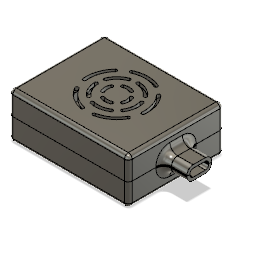
GBIP-uno (Autodesk Fusion 360 design; units mm, degrees)
Autodesk Fusion 360 part; units mm, degrees
sketch "Sketch1" plane through (0, 0, 0) normal (0, 1, 0) x (1, 0, 0)
  line L0 (0, 53.2694) -> (68.6417, 53.2694)
  line L1 (68.6417, 53.2694) -> (68.6417, 0.0072)
  line L2 (68.6417, 0.0072) -> (0, 0.0072)
  line L3 (0, 0.0072) -> (0, 53.2694)
  line L4 (70.6417, -1.9928) -> (-2, -1.9928)
  line L5 (-2, -1.9928) -> (-2, 55.2694)
  line L6 (-2, 55.2694) -> (70.6417, 55.2694)
  line L7 (70.6417, 55.2694) -> (70.6417, -1.9928)
  line L8 (70.1417, -4.4928) -> (-1.5, -4.4928)
  line L9 (-4.5, -1.4928) -> (-4.5, 54.7694)
  line L10 (-1.5, 57.7694) -> (70.1417, 57.7694)
  line L11 (73.1417, 54.7694) -> (73.1417, -1.4928)
  arc A0 (-1.5, 57.7694) -> (-4.5, 54.7694) centre (-1.5, 54.7694) ccw
  arc A1 (73.1417, 54.7694) -> (70.1417, 57.7694) centre (70.1417, 54.7694) ccw
  arc A2 (70.1417, -4.4928) -> (73.1417, -1.4928) centre (70.1417, -1.4928) ccw
  arc A3 (-4.5, -1.4928) -> (-1.5, -4.4928) centre (-1.5, -1.4928) ccw
  line L12 (11.9, 3.5) -> (0, 3.5)
  line L13 (0, 3.5) -> (0, 0)
  line L14 (0, 0) -> (66.1, 0)
  line L15 (66.1, 0) -> (66.1, 2)
  line L16 (66.1, 2) -> (68.6, 4.5)
  line L17 (68.6, 4.5) -> (68.6, 37.8)
  line L18 (68.6, 37.8) -> (66.1, 40.3)
  line L19 (66.1, 40.3) -> (66.1, 53.3)
  line L20 (66.1, 53.3) -> (0, 53.3)
  line L21 (0, 53.3) -> (0, 44)
  line L22 (0, 44) -> (10.1, 44)
  line L23 (10.1, 44) -> (10.1, 31.6)
  line L24 (10.1, 31.6) -> (0, 31.6)
  line L25 (0, 31.6) -> (0, 12.4)
  line L26 (0, 12.4) -> (11.9, 12.4)
  line L27 (11.9, 12.4) -> (11.9, 3.5)
  circle A4 centre (14, 2.5) radius 1.6
  circle A5 centre (15.3, 50.7) radius 1.6
  circle A6 centre (66.1, 35.5) radius 1.6
  circle A7 centre (66.1, 7.6) radius 1.6
  dimension "d13" = -2
  dimension "d15" = 3
  dimension "d16" = 3
  dimension "d17" = 3
  dimension "d18" = 3
  constraint horizontal L0
  constraint vertical L1
  constraint horizontal L2
  constraint vertical L3
  constraint parallel L2 L8
  constraint parallel L3 L9
  constraint parallel L0 L10
  constraint parallel L1 L11
  constraint tangent L10 A0
  constraint tangent L9 A0
  constraint tangent L10 A1
  constraint tangent L11 A1
  constraint tangent L11 A2
  constraint tangent L8 A2
  constraint tangent L8 A3
  constraint tangent L9 A3
  measures "d15" radius of A0
  measures "d16" radius of A1
  measures "d17" radius of A2
  measures "d18" radius of A3
sketch "Sketch2" plane through (0, 0, 0) normal (0, 1, 0) x (1, 0, 0)
box "BoxPrimitive1" add length 57.2712 width 72.6733 height 25 placed x (0, 0, -1) y (-1, 0, 0) z (0, 1, 0) at (70.6572, 0, 1.9989) makes body 1
shell "Shell1" thickness 2.2 outward yes removed faces 0 bodies 1
fillet "Fillet1" radius 2.5 6 faces at (47.1662, 27.2, -36.9153) (72.8572, 7.6, -36.9153) (47.1662, 7.6, 4.1989) (-4.216, 7.6, -36.9153) (47.1662, 7.6, -57.4724) (47.1662, -2.2, -36.9153) on bodies 1
ref_plane "WorkPlane1" through (34.3206, 12.5, -26.6367) normal (0, 1, 0) x (0, 0, -1)
split "Split1" by plane through (34.3206, 12.5, -26.6367) normal (0, 1, 0) bodies 1 makes body 2 at (46.4328, 25, -36.182)
sketch "Sketch4" plane through (0, 0, 0) normal (0, 1, 0) x (-1, 0, 0)
  line L0 (-70.6572, -55.2724) -> (2.016, -55.2724)
  line L1 (2.016, -55.2724) -> (2.016, 1.9989)
  line L2 (2.016, 1.9989) -> (-70.6572, 1.9989)
  line L3 (-70.6572, 1.9989) -> (-70.6572, -55.2724)
  line L4 (-11.9, -3.5) -> (0, -3.5)
  line L5 (0, -3.5) -> (0, 0)
  line L6 (0, 0) -> (-66.1, 0)
  line L7 (-66.1, 0) -> (-66.1, -2)
  line L8 (-66.1, -2) -> (-68.6, -4.5)
  line L9 (-68.6, -4.5) -> (-68.6, -37.8)
  line L10 (-68.6, -37.8) -> (-66.1, -40.3)
  line L11 (-66.1, -40.3) -> (-66.1, -53.3)
  line L12 (-66.1, -53.3) -> (0, -53.3)
  line L13 (0, -53.3) -> (0, -44)
  line L14 (0, -44) -> (-10.1, -44)
  line L15 (-10.1, -44) -> (-10.1, -31.6)
  line L16 (-10.1, -31.6) -> (0, -31.6)
  line L17 (0, -31.6) -> (0, -12.4)
  line L18 (0, -12.4) -> (-11.9, -12.4)
  line L19 (-11.9, -12.4) -> (-11.9, -3.5)
  circle A0 centre (-14, -2.5) radius 1.6
  circle A1 centre (-15.3, -50.7) radius 1.6
  circle A2 centre (-66.1, -35.5) radius 1.6
  circle A3 centre (-66.1, -7.6) radius 1.6
sketch "Sketch5" plane through (0, 5.6, 0) normal (0, 1, 0) x (-1, 0, 0)
  line L0 (-11.9, -3.5) -> (0, -3.5)
  line L1 (0, -3.5) -> (0, 0)
  line L2 (0, 0) -> (-66.1, 0)
  line L3 (-66.1, 0) -> (-66.1, -2)
  line L4 (-66.1, -2) -> (-68.6, -4.5)
  line L5 (-68.6, -4.5) -> (-68.6, -37.8)
  line L6 (-68.6, -37.8) -> (-66.1, -40.3)
  line L7 (-66.1, -40.3) -> (-66.1, -53.3)
  line L8 (-66.1, -53.3) -> (0, -53.3)
  line L9 (0, -53.3) -> (0, -44)
  line L10 (0, -44) -> (-10.1, -44)
  line L11 (-10.1, -44) -> (-10.1, -31.6)
  line L12 (-10.1, -31.6) -> (0, -31.6)
  line L13 (0, -31.6) -> (0, -12.4)
  line L14 (0, -12.4) -> (-11.9, -12.4)
  line L15 (-11.9, -12.4) -> (-11.9, -3.5)
  circle A0 centre (-14, -2.5) radius 1.6
  circle A1 centre (-15.3, -50.7) radius 1.6
  circle A2 centre (-66.1, -35.5) radius 1.6
  circle A3 centre (-66.1, -7.6) radius 1.6
  circle A4 centre (-15.3, -50.7) radius 2
  circle A5 centre (-66.1, -35.5) radius 2
  circle A6 centre (-14, -2.5) radius 2
  circle A7 centre (-66.1, -7.6) radius 2
  dimension "d30" = 4
  dimension "d31" = 4
  dimension "d32" = 4
  dimension "d33" = 4
  constraint concentric A1 A4
  constraint concentric A2 A5
  constraint concentric A0 A6
  constraint concentric A3 A7
  measures "d30" diameter of A4
  measures "d31" diameter of A5
  measures "d32" diameter of A6
  measures "d33" diameter of A7
extrude "Extrude1" add sketch "Sketch4" along normal blind 4 contours A0 | A1 | A2 | A3 bodies 1
ref_plane "WorkPlane2" through (16.9, 4, -50.7) normal (0, -1, 0) x (1, 0, 0)
sketch "Sketch6" plane through (16.9, 4, -50.7) normal (0, -1, 0) x (1, 0, 0)
  line L0 (-5, 47.2) -> (-16.9, 47.2)
  line L1 (-16.9, 47.2) -> (-16.9, 50.7)
  line L2 (-16.9, 50.7) -> (49.2, 50.7)
  line L3 (49.2, 50.7) -> (49.2, 48.7)
  line L4 (49.2, 48.7) -> (51.7, 46.2)
  line L5 (51.7, 46.2) -> (51.7, 12.9)
  line L6 (51.7, 12.9) -> (49.2, 10.4)
  line L7 (49.2, 10.4) -> (49.2, -2.6)
  line L8 (49.2, -2.6) -> (-16.9, -2.6)
  line L9 (-16.9, -2.6) -> (-16.9, 6.7)
  line L10 (-16.9, 6.7) -> (-6.8, 6.7)
  line L11 (-6.8, 6.7) -> (-6.8, 19.1)
  line L12 (-6.8, 19.1) -> (-16.9, 19.1)
  line L13 (-16.9, 19.1) -> (-16.9, 38.3)
  line L14 (-16.9, 38.3) -> (-5, 38.3)
  line L15 (-5, 38.3) -> (-5, 47.2)
  circle A0 centre (-2.9, 48.2) radius 1.6
  circle A1 centre (-1.6, 0) radius 1.6
  circle A2 centre (49.2, 15.2) radius 1.6
  circle A3 centre (49.2, 43.1) radius 1.6
  circle A4 centre (-1.6, 0) radius 1.5
  circle A5 centre (49.2, 15.2) radius 1.5
  circle A6 centre (49.2, 43.1) radius 1.5
  circle A7 centre (-2.9, 48.2) radius 1.5
  dimension "d36" = 3
  dimension "d37" = 3
  dimension "d38" = 3
  dimension "d39" = 3
  constraint concentric A1 A4
  constraint concentric A2 A5
  constraint concentric A3 A6
  constraint concentric A0 A7
  measures "d36" diameter of A4
  measures "d37" diameter of A5
  measures "d38" diameter of A6
  measures "d39" diameter of A7
extrude "Extrude2" add sketch "Sketch6" against normal blind 12 contours A4 | A5 | A6 | A7 bodies 1
fillet "Fillet2" radius 1 4 edges at (12.6015, 16, -1.9576) (13.9015, 16, -50.1576) (64.7015, 16, -34.9576) (64.7015, 16, -7.0576) on bodies 1
fillet "Fillet3" radius 2 4 edges at (16.7917, 0, -50.1214) (15.4917, 0, -1.9214) (67.5917, 0, -7.0214) (67.5917, 0, -34.9214) on bodies 1
sketch "Sketch7" plane through (0, 25, 0) normal (0, -1, 0) x (1, 0, 0)
  line L0 (-2.016, -55.2724) -> (70.6572, -55.2724)
  line L1 (70.6572, -55.2724) -> (70.6572, 1.9989)
  line L2 (70.6572, 1.9989) -> (-2.016, 1.9989)
  line L3 (-2.016, 1.9989) -> (-2.016, -55.2724)
  circle A0 centre (13.8798, -3.0788) radius 1.6
  circle A1 centre (65.9798, -8.1788) radius 1.6
  circle A2 centre (65.9798, -36.0788) radius 1.6
  circle A3 centre (15.1798, -51.2788) radius 1.6
  line L4 (-0.1202, -44.5788) -> (-0.1202, -32.1788)
  line L5 (-0.1202, -32.1788) -> (-6.4202, -32.1788)
  line L6 (-6.4202, -32.1788) -> (-6.4202, -44.5788)
  line L7 (-6.4202, -44.5788) -> (-0.1202, -44.5788)
  line L8 (-2.4202, -12.9788) -> (-0.1202, -12.9788)
  line L9 (-0.1202, -12.9788) -> (-0.1202, -4.0788)
  line L10 (-0.1202, -4.0788) -> (-2.4202, -4.0788)
  line L11 (-2.4202, -4.0788) -> (-2.4202, -12.9788)
  line L12 (-2.4202, -12.9788) -> (-0.1202, -12.9788)
sketch "Sketch8" plane through (0, 25, 0) normal (0, -1, 0) x (1, 0, 0)
  circle A0 centre (13.8798, -3.0788) radius 2.1
  circle A1 centre (13.8798, -3.0788) radius 1.6
  circle A2 centre (65.9798, -8.1788) radius 2.1
  circle A3 centre (65.9798, -8.1788) radius 1.6
  circle A4 centre (15.1798, -51.2788) radius 2.1
  circle A5 centre (15.1798, -51.2788) radius 1.6
  circle A6 centre (65.9798, -36.0788) radius 2.1
  circle A7 centre (65.9798, -36.0788) radius 1.6
  point P0 (13.8798, -3.0788)
  point P1 (65.9798, -8.1788)
  point P2 (15.1798, -51.2788)
  point P3 (65.9798, -36.0788)
  dimension "d46" = 4.2
  dimension "d47" = 3.2
  dimension "d48" = 4.2
  dimension "d49" = 3.2
  dimension "d50" = 4.2
  dimension "d51" = 3.2
  dimension "d52" = 4.2
  dimension "d53" = 3.2
  constraint coincident P0 A0.centre
  constraint coincident P1 A2.centre
  constraint concentric A2 A3
  constraint coincident P2 A4.centre
  constraint concentric A4 A5
  constraint coincident P3 A6.centre
  constraint concentric A6 A7
  measures "d46" diameter of A0
  measures "d47" diameter of A1
  measures "d48" diameter of A2
  measures "d49" diameter of A3
  measures "d50" diameter of A4
  measures "d51" diameter of A5
  measures "d52" diameter of A6
  measures "d53" diameter of A7
extrude "Extrude3" add sketch "Sketch8" along normal blind 12 bodies 2
fillet "Fillet4" radius 2 4 edges at (11.9219, 25, -2.3194) (64.0219, 25, -7.4194) (64.0219, 25, -35.3194) (13.2219, 25, -50.5194) on bodies 2
sketch "Sketch9" plane through (-4.216, 0, 0) normal (-1, 0, 0) x (0, 0, 1)
  line L0 (1.6989, 12.5) -> (-54.9724, 12.5)
  line L1 (-54.9724, 12.5) -> (-54.9724, 0.3)
  line L2 (-54.9724, 0.3) -> (1.6989, 0.3)
  line L3 (1.6989, 0.3) -> (1.6989, 12.5)
  line L4 (-44.5788, 6.3999) -> (-32.1788, 6.3999)
  line L5 (-32.1788, 6.3999) -> (-32.1788, 17.2999)
  line L6 (-32.1788, 17.2999) -> (-44.5788, 17.2999)
  line L7 (-44.5788, 17.2999) -> (-44.5788, 6.3999)
  line L8 (-12.9788, 6.3999) -> (-4.0788, 6.3999)
  line L9 (-4.0788, 6.3999) -> (-4.0788, 17.1999)
  line L10 (-4.0788, 17.1999) -> (-12.9788, 17.1999)
  line L11 (-12.9788, 17.1999) -> (-12.9788, 6.3999)
  line L12 (-31.1788, 5.3999) -> (-31.1788, 18.2999)
  line L13 (-31.1788, 18.2999) -> (-45.5788, 18.2999)
  line L14 (-45.5788, 18.2999) -> (-45.5788, 5.3999)
  line L15 (-45.5788, 5.3999) -> (-31.1788, 5.3999)
  line L16 (-3.0788, 5.3999) -> (-3.0788, 18.1999)
  line L17 (-3.0788, 18.1999) -> (-13.9788, 18.1999)
  line L18 (-13.9788, 18.1999) -> (-13.9788, 5.3999)
  line L19 (-13.9788, 5.3999) -> (-3.0788, 5.3999)
  dimension "d58" = 1
  dimension "d59" = 1
extrude "Extrude4" cut sketch "Sketch9" against normal blind 4 contours L0 L8 L9 L11 L16 L18 L19 | L0 L8 L9 L11 | L0 L4 L5 L7 L12 L14 L15 | L0 L4 L5 L7 bodies 1
sketch "Sketch10" plane through (-4.216, 0, 0) normal (-1, 0, 0) x (0, 0, 1)
  line L0 (-54.9724, 12.5) -> (1.6989, 12.5)
  line L1 (1.6989, 12.5) -> (1.6989, 24.7)
  line L2 (1.6989, 24.7) -> (-54.9724, 24.7)
  line L3 (-54.9724, 24.7) -> (-54.9724, 12.5)
  line L4 (-44.5788, 6.3999) -> (-32.1788, 6.3999)
  line L5 (-32.1788, 6.3999) -> (-32.1788, 17.2999)
  line L6 (-32.1788, 17.2999) -> (-44.5788, 17.2999)
  line L7 (-44.5788, 17.2999) -> (-44.5788, 6.3999)
  line L8 (-12.9788, 6.3999) -> (-4.0788, 6.3999)
  line L9 (-4.0788, 6.3999) -> (-4.0788, 17.1999)
  line L10 (-4.0788, 17.1999) -> (-12.9788, 17.1999)
  line L11 (-12.9788, 17.1999) -> (-12.9788, 6.3999)
  line L12 (-45.5788, 18.2999) -> (-45.5788, 5.3999)
  line L13 (-45.5788, 5.3999) -> (-31.1788, 5.3999)
  line L14 (-31.1788, 5.3999) -> (-31.1788, 18.2999)
  line L15 (-31.1788, 18.2999) -> (-45.5788, 18.2999)
  line L16 (-3.0788, 5.3999) -> (-3.0788, 18.1999)
  line L17 (-3.0788, 18.1999) -> (-13.9788, 18.1999)
  line L18 (-13.9788, 18.1999) -> (-13.9788, 5.3999)
  line L19 (-13.9788, 5.3999) -> (-3.0788, 5.3999)
  dimension "d62" = 1
  dimension "d63" = 1
extrude "Extrude5" cut sketch "Sketch10" against normal blind 4 contours L0 L5 L6 L7 L12 L14 L15 | L0 L5 L6 L7 | L0 L9 L10 L11 L16 L17 L18 | L0 L9 L10 L11 bodies 2
sketch "Sketch11" plane through (72.8572, 0, 0) normal (1, 0, 0) x (0, 0, -1)
  line L0 (-1.6989, 12.5) -> (54.9724, 12.5)
  line L1 (54.9724, 12.5) -> (54.9724, 24.7)
  line L2 (54.9724, 24.7) -> (-1.6989, 24.7)
  line L3 (-1.6989, 24.7) -> (-1.6989, 12.5)
  line L4 (30.6367, 15) -> (22.6367, 15)
  line L5 (20.6367, 13) -> (20.6367, 12)
  line L6 (22.6367, 10) -> (30.6367, 10)
  line L7 (32.6367, 12) -> (32.6367, 13)
  line L8 (32.6367, 15) -> (20.6367, 10) construction
  line L9 (20.6367, 15) -> (32.6367, 10) construction
  arc A0 (22.6367, 15) -> (20.6367, 13) centre (22.6367, 13) ccw
  arc A1 (32.6367, 13) -> (30.6367, 15) centre (30.6367, 13) ccw
  arc A2 (20.6367, 12) -> (22.6367, 10) centre (22.6367, 12) ccw
  arc A3 (30.6367, 10) -> (32.6367, 12) centre (30.6367, 12) ccw
  line L10 (18.6367, 13) -> (18.6367, 12)
  arc A4 (18.6367, 12) -> (22.6367, 8) centre (22.6367, 12) ccw
  line L11 (22.6367, 8) -> (30.6367, 8)
  arc A5 (30.6367, 8) -> (34.6367, 12) centre (30.6367, 12) ccw
  line L12 (34.6367, 12) -> (34.6367, 13)
  arc A6 (34.6367, 13) -> (30.6367, 17) centre (30.6367, 13) ccw
  line L13 (30.6367, 17) -> (22.6367, 17)
  arc A7 (22.6367, 17) -> (18.6367, 13) centre (22.6367, 13) ccw
  point P0 (26.6367, 12.5)
  dimension "d66" = 12
  dimension "d67" = 5
  dimension "d68" = 2
  dimension "d69" = 2
  dimension "d70" = 2
  dimension "d71" = 2
  dimension "d72" = 2
  constraint horizontal L4
  constraint perpendicular L4 L5
  constraint parallel L4 L6
  constraint parallel L5 L7
  constraint coincident L8 P0
  constraint coincident L9 P0
  constraint midpoint L0 P0
  constraint coincident L9.start L4
  constraint coincident L9.start L5
  constraint tangent L4 A0
  constraint tangent L5 A0
  constraint coincident L8.start L4
  constraint coincident L8.start L7
  constraint tangent L4 A1
  constraint tangent L7 A1
  constraint coincident L8.end L5
  constraint coincident L8.end L6
  constraint tangent L5 A2
  constraint tangent L6 A2
  constraint coincident L9.end L6
  constraint coincident L9.end L7
  constraint tangent L6 A3
  constraint tangent L7 A3
  measures "d66" distance of L8.end L9.end
  measures "d67" distance of L9.start L8.end
  measures "d68" radius of A0
  measures "d69" radius of A1
  measures "d70" radius of A2
  measures "d71" radius of A3
extrude "Extrude6" add sketch "Sketch11" along normal blind 15 contours L0 L5 L6 L7 A2 A3 L10 A4 L11 A5 L12 bodies 1
extrude "Extrude7" cut 1 faces at (72.8572, 11.6667, -27.9701) along direction (-1, 0, 0) blind 5 on bodies 1 bodies 1
extrude "Extrude8" add sketch "Sketch11" along normal blind 15 contours L0 L4 L5 L7 A0 A1 L10 L12 A6 L13 A7 bodies 2
extrude "Extrude9" cut sketch "Sketch11" against normal blind 5 contours L0 L4 L5 L7 A0 A1 bodies 2
fillet "Fillet7" radius 5 5 edges at (72.8572, 12.75, -18.6367) (72.8572, 15.8284, -19.8083) (72.8572, 17, -26.6367) (72.8572, 15.8284, -33.4652) (72.8572, 12.75, -34.6367) on bodies 2
fillet "Fillet8" radius 5 5 edges at (72.8572, 12.25, -34.6367) (72.8572, 9.1716, -33.4652) (72.8572, 8, -26.6367) (72.8572, 9.1716, -19.8083) (72.8572, 12.25, -18.6367) on bodies 1
sketch "Sketch12" plane through (0, 27.2, 0) normal (0, 1, 0) x (-1, 0, 0)
  line L0 (-70.3572, -54.9724) -> (1.716, -54.9724)
  line L1 (1.716, -54.9724) -> (1.716, 1.6989)
  line L2 (1.716, 1.6989) -> (-70.3572, 1.6989)
  line L3 (-70.3572, 1.6989) -> (-70.3572, -54.9724)
  arc A0 (-52.0597, -25.1523) -> (-54.0463, -24.9216) centre (-53.053, -25.0369) ccw
  arc A1 (-30.9479, -15.6722) -> (-40.8248, -17.2365) centre (-34.1798, -27.2288) ccw
  arc A2 (-30.4092, -13.7461) -> (-41.9323, -15.5711) centre (-34.1798, -27.2288) ccw
  arc A3 (-21.0558, -32.1032) -> (-22.9307, -31.4068) centre (-21.9932, -31.755) ccw
  arc A4 (-43.5873, -34.6785) -> (-45.1552, -35.9202) centre (-44.3713, -35.2993) ccw
  arc A5 (-41.6798, -43.5918) -> (-42.5132, -45.4099) centre (-42.0965, -44.5009) ccw
  arc A6 (-25.8465, -45.4099) -> (-26.6798, -43.5918) centre (-26.2632, -44.5009) ccw
  arc A7 (-44.1721, -20.5838) -> (-45.8374, -19.4763) centre (-45.0047, -20.0301) ccw
  arc A8 (-39.6342, -24.7288) -> (-41.465, -23.9234) centre (-40.5867, -24.4104) ccw
  arc A9 (-30.8744, -19.9435) -> (-37.4852, -19.9435) centre (-34.1798, -27.2288) ccw
  arc A10 (-31.6798, -21.7744) -> (-36.6798, -21.7744) centre (-34.1798, -27.2288) ccw
  arc A11 (-26.8946, -23.9234) -> (-28.7255, -24.7288) centre (-27.7729, -24.4104) ccw
  arc A12 (-25.4884, -16.2534) -> (-26.73, -17.8213) centre (-26.1092, -17.0373) ccw
  arc A13 (-14.3134, -24.9216) -> (-16.3, -25.1523) centre (-15.3067, -25.0369) ccw
  arc A14 (-37.7302, -9.5824) -> (-38.1247, -7.6217) centre (-37.9274, -8.602) ccw
  arc A15 (-30.235, -7.6217) -> (-30.6295, -9.5824) centre (-30.4322, -8.602) ccw
  arc A16 (-36.6798, -32.6831) -> (-37.4852, -34.514) centre (-36.9982, -33.6356) ccw
  arc A17 (-30.8744, -34.514) -> (-31.6798, -32.6831) centre (-31.3615, -33.6356) ccw
  arc A18 (-18.4942, -18.3991) -> (-30.6295, -9.5824) centre (-34.1798, -27.2288) ccw
  arc A19 (-18.4942, -18.3991) -> (-16.7514, -17.4181) centre (-17.6228, -17.9086) ccw
  arc A20 (-16.7514, -17.4181) -> (-30.235, -7.6217) centre (-34.1798, -27.2288) ccw
  arc A21 (-52.0597, -25.1523) -> (-47.4244, -39.4181) centre (-34.1798, -27.2288) ccw
  arc A22 (-54.0463, -24.9216) -> (-48.896, -40.7725) centre (-34.1798, -27.2288) ccw
  arc A23 (-48.896, -40.7725) -> (-47.4244, -39.4181) centre (-48.1602, -40.0953) ccw
  arc A24 (-22.1901, -26.7313) -> (-26.73, -17.8213) centre (-34.1798, -27.2288) ccw
  arc A25 (-22.1901, -26.7313) -> (-20.1919, -26.6484) centre (-21.191, -26.6899) ccw
  arc A26 (-20.1919, -26.6484) -> (-25.4884, -16.2534) centre (-34.1798, -27.2288) ccw
  arc A27 (-31.6798, -21.7744) -> (-30.8744, -19.9435) centre (-31.3615, -20.8219) ccw
  arc A28 (-37.4852, -19.9435) -> (-36.6798, -21.7744) centre (-36.9982, -20.8219) ccw
  arc A29 (-47.6625, -30.9994) -> (-45.7364, -30.4607) centre (-46.6995, -30.73) ccw
  arc A30 (-44.1721, -20.5838) -> (-45.7364, -30.4607) centre (-34.1798, -27.2288) ccw
  arc A31 (-45.8374, -19.4763) -> (-47.6625, -30.9994) centre (-34.1798, -27.2288) ccw
  arc A32 (-34.7602, -41.2167) -> (-34.6772, -39.2184) centre (-34.7187, -40.2176) ccw
  arc A33 (-43.5873, -34.6785) -> (-34.6772, -39.2184) centre (-34.1798, -27.2288) ccw
  arc A34 (-45.1552, -35.9202) -> (-34.7602, -41.2167) centre (-34.1798, -27.2288) ccw
  arc A35 (-41.9323, -15.5711) -> (-40.8248, -17.2365) centre (-41.3785, -16.4038) ccw
  arc A36 (-30.9479, -15.6722) -> (-30.4092, -13.7461) centre (-30.6786, -14.7091) ccw
  arc A37 (-30.0017, -38.4779) -> (-22.9307, -31.4068) centre (-34.1798, -27.2288) ccw
  arc A38 (-30.0017, -38.4779) -> (-29.3054, -40.3528) centre (-29.6536, -39.4153) ccw
  arc A39 (-29.3054, -40.3528) -> (-21.0558, -32.1032) centre (-34.1798, -27.2288) ccw
  arc A40 (-41.6798, -43.5918) -> (-26.6798, -43.5918) centre (-34.1798, -27.2288) ccw
  arc A41 (-42.5132, -45.4099) -> (-25.8465, -45.4099) centre (-34.1798, -27.2288) ccw
  arc A42 (-39.6342, -24.7288) -> (-39.6342, -29.7288) centre (-34.1798, -27.2288) ccw
  arc A43 (-41.465, -23.9234) -> (-41.465, -30.5341) centre (-34.1798, -27.2288) ccw
  arc A44 (-41.465, -30.5341) -> (-39.6342, -29.7288) centre (-40.5867, -30.0471) ccw
  arc A45 (-28.7255, -29.7288) -> (-28.7255, -24.7288) centre (-34.1798, -27.2288) ccw
  arc A46 (-28.7255, -29.7288) -> (-26.8946, -30.5341) centre (-27.7729, -30.0471) ccw
  arc A47 (-26.8946, -30.5341) -> (-26.8946, -23.9234) centre (-34.1798, -27.2288) ccw
  arc A48 (-20.9353, -39.4181) -> (-16.3, -25.1523) centre (-34.1798, -27.2288) ccw
  arc A49 (-20.9353, -39.4181) -> (-19.4636, -40.7725) centre (-20.1994, -40.0953) ccw
  arc A50 (-19.4636, -40.7725) -> (-14.3134, -24.9216) centre (-34.1798, -27.2288) ccw
  arc A51 (-37.7302, -9.5824) -> (-49.8654, -18.3991) centre (-34.1798, -27.2288) ccw
  arc A52 (-38.1247, -7.6217) -> (-51.6083, -17.4181) centre (-34.1798, -27.2288) ccw
  arc A53 (-51.6083, -17.4181) -> (-49.8654, -18.3991) centre (-50.7368, -17.9086) ccw
  arc A54 (-36.6798, -32.6831) -> (-31.6798, -32.6831) centre (-34.1798, -27.2288) ccw
  arc A55 (-37.4852, -34.514) -> (-30.8744, -34.514) centre (-34.1798, -27.2288) ccw
  line L4 (-66.4798, -56.4788) -> (-1.8798, -56.4788)
  line L5 (-71.0798, -2.5788) -> (-71.0798, -51.8788)
  line L6 (-1.8798, 2.0212) -> (-66.4798, 2.0212)
  line L7 (2.7202, -51.8788) -> (2.7202, -2.5788)
  arc A56 (2.7202, -2.5788) -> (-1.8798, 2.0212) centre (-1.8798, -2.5788) ccw
  arc A57 (-1.8798, -56.4788) -> (2.7202, -51.8788) centre (-1.8798, -51.8788) ccw
  arc A58 (-66.4798, 2.0212) -> (-71.0798, -2.5788) centre (-66.4798, -2.5788) ccw
  arc A59 (-71.0798, -51.8788) -> (-66.4798, -56.4788) centre (-66.4798, -51.8788) ccw
extrude "Extrude10" cut sketch "Sketch12" against normal blind 3 contours A0 A21 A22 A23 | A1 A2 A35 A36 | A3 A37 A38 A39 | A4 A32 A33 A34 | A5 A6 A40 A41 | A7 A29 A30 A31 | A8 A42 A43 A44 | A9 A10 A27 A28 | A11 A45 A46 A47 | A12 A24 A25 A26 | A13 A48 A49 A50 | A14 A51 A52 A53 | A15 A18 A19 A20 | A16 A17 A54 A55 bodies 2
fillet "Fillet5" [suppressed]
fillet "Fillet6" [suppressed]
named bodies: "uno_bottom", "uno_top"
